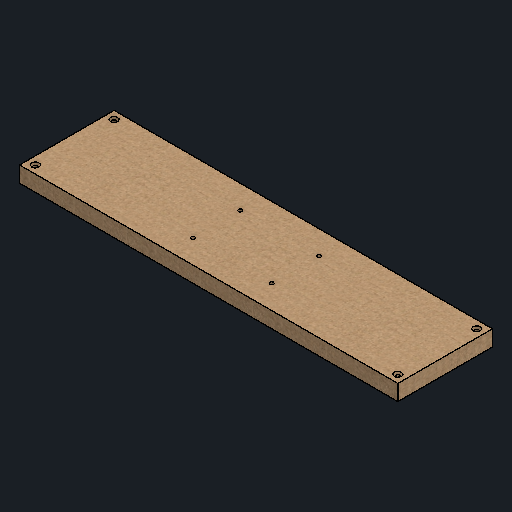
# Autodesk Inventor part: Part3
Saved by Autodesk Inventor 2026.2 (Build 302298000, 298)
## iProperties
Created: 2026-06-15
Part Number: Part3
Material: MDF Medium Density Fiberboard
Document SubType Name: Modeling
Designer: JoshuaEah
Density: 0.8 g/cm^3
Appearance: Cardboard - Corrugated
Author: JoshuaEah
Autodesk Inventor part; units mm, degrees
ref_plane "YZ Plane" through (0, 0, 0) normal (1, 0, 0) x (0, 1, 0)
ref_plane "XZ Plane" through (0, 0, 0) normal (0, 1, 0) x (-1, 0, 0)
ref_plane "XY Plane" through (0, 0, 0) normal (0, 0, 1) x (1, 0, 0)
sketch "Sketch1" plane through (0, 0, 0) normal (0, 1, 0) x (-1, 0, 0)
  line L0 (0, 0) -> (-304.8, 0)
  line L1 (-304.8, 0) -> (-304.8, -76.2)
  line L2 (-304.8, -76.2) -> (0, -76.2)
  line L3 (0, -76.2) -> (0, 0)
  line L4 (0, -38.1) -> (-304.8, -38.1)
  line L5 (-152.4, -76.2) -> (-152.4, 0)
  point P0 (-6.35, -69.85)
  point P1 (-6.35, -6.35)
  point P2 (-298.45, -69.85)
  point P3 (-298.45, -6.35)
  dimension "d0" = 76.2
  dimension "d1" = 304.8
  dimension "d17" = 6.35
  dimension "d18" = 6.35
  constraints: 12 end point, 4 midpoint, 3 symmetric about line, 2 parallel, 1 coincident, 1 horizontal, 1 perpendicular
  measures "d0" distance of L2.end L0.start
  measures "d1" distance of L0.start L0.end
  measures "d17" distance from line of L3 point (-6.35, -69.85)
  measures "d18" distance from line of L2 point (-6.35, -69.85)
extrude "Extrusion1" add sketch "Sketch1" against normal blind 12.7
hole "Back Panel Mount Hole" at (6.35, 0, -69.85) direction (0, -1, 0) diameter 3.2766 end through all start extended yes countersink diameter 5.715 countersink angle 82 clearance for "Flat Head Machine Screw (82)" size "#4" standard "Ansi Unified Screw Threads"
pattern_sketch "Back Panel Mounting Holes" of "Back Panel Mount Hole" from (6.35, 0, -69.85) copies at (6.35, 0, -6.35) at (298.45, 0, -69.85) at (298.45, 0, -6.35)
sketch "Name Plate Hole Pattern" plane through (0, 0, 0) normal (0, 1, 0) x (1, 0, 0)
  line L0 (127, 25.4) -> (177.8, 25.4) construction
  line L1 (177.8, 25.4) -> (177.8, 50.8) construction
  line L2 (177.8, 50.8) -> (127, 50.8) construction
  line L3 (127, 50.8) -> (127, 25.4) construction
  line L4 (127, 25.4) -> (177.8, 50.8) construction
  line L5 (177.8, 25.4) -> (127, 50.8) construction
  line L6 (152.4, 76.2) -> (152.4, 0) projected
  line L7 (184.15, 19.05) -> (120.65, 19.05) construction
  line L8 (120.65, 19.05) -> (120.65, 57.15) construction
  line L9 (120.65, 57.15) -> (184.15, 57.15) construction
  line L10 (184.15, 57.15) -> (184.15, 19.05) construction
  point P0 (152.4, 38.1)
  dimension "d19" = 50.8
  dimension "d20" = 25.4
  dimension "d21" = 6.35
  constraints: 20 end point, 4 coincident, 4 parallel, 3 midpoint, 2 perpendicular, 1 horizontal, 3 other
  measures "d19" distance of L2.end L1.end
  measures "d20" distance of L1.end L0.end
  measures "d21" distance between parallel lines of L0 L7
hole "Name Plate Mounting Hole" at (120.65, 0, -57.15) direction (0, -1, 0) diameter 2.9464 end through all start extended yes clearance for "Flat Head Machine Screw (82)" size "#4" standard "Ansi Unified Screw Threads"
pattern_sketch "Name Plate Mounting Holes" of "Name Plate Mounting Hole" from (120.65, 0, -57.15) copies at (184.15, 0, -57.15) at (184.15, 0, -19.05) at (120.65, 0, -19.05)
equation "\"d18\" = d17"
body "Solid1"
